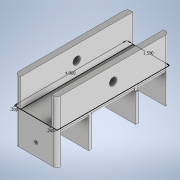
# Autodesk Inventor part: Sample Holder end for 8020-thruhole-widestance-long
Saved by Autodesk Inventor 2020 (Build 240168000, 168)
## iProperties
Created: 2022-02-15
Part Number: Sample Holder end for 8020-thruhole-widestance-long
Material: Generic
Document SubType Name: Modeling
Designer: Beaucage
Density: 1 g/cm^3
Appearance: Default
Author: Beaucage
Autodesk Inventor part; units mm, degrees
ref_plane "YZ Plane" through (0, 0, 0) normal (1, 0, 0) x (0, 1, 0)
ref_plane "XZ Plane" through (0, 0, 0) normal (0, 1, 0) x (-1, 0, 0)
ref_plane "XY Plane" through (0, 0, 0) normal (0, 0, 1) x (1, 0, 0)
sketch "Sketch1" plane through (0, 0, 0) normal (0, 1, 0) x (-1, 0, 0)
  line L0 (0, 0) -> (38.1, 0)
  line L1 (38.1, 0) -> (38.1, -101.6)
  line L2 (38.1, -101.6) -> (0, -101.6)
  line L3 (0, -101.6) -> (0, 0)
  line L4 (38.1, -101.6) -> (33.02, -101.6)
  line L5 (33.02, -101.6) -> (33.02, 0)
  line L6 (33.02, 0) -> (38.1, 0)
  line L7 (38.1, 0) -> (38.1, -101.6)
  line L8 (0, -101.6) -> (5.08, -101.6)
  line L9 (5.08, -101.6) -> (5.08, 0)
  line L10 (5.08, 0) -> (0, 0)
  line L11 (0, 0) -> (0, -101.6)
  dimension "d0" = 38.1
  dimension "d1" = 101.6
  dimension "d2" = 5.08
  dimension "d3" = 5.08
  constraints: 24 end point, 6 parallel, 3 horizontal, 3 perpendicular, 2 point on line
  measures "d0" distance of L1.end L2.end
  measures "d1" distance of L0.end L1.end
  measures "d2" distance of L5.end L6.end
  measures "d3" distance of L10.end L9.end
extrude "Extrusion1" add sketch "Sketch1" along normal blind 25.4 contours L0 L9 L2 L3 | L0 L1 L2 L5
extrude "Extrusion2" add sketch "Sketch1" against normal blind 5.08
sketch "Sketch2" plane through (0, 25.4, 0) normal (1, 0, 0) x (0, 0, -1)
  line L0 (101.6, 0) -> (0, 0) projected
  line L1 (50.8, 0) -> (50.8, -12.7)
  point P0 (0, -25.4)
  dimension "d8" = 12.7
  constraints: 2 end point, 1 midpoint, 1 vertical
  measures "d8" distance of L1.start L1.end
hole "Hole1" at (0, 12.7, -50.8) direction (-1, 0, 0) diameter 6.7564 end through all clearance for "Socket Head Cap Screw" size "1/4" standard "Ansi Unified Screw Threads"
sketch "Sketch3" plane through (0, -5.08, 0) normal (0, -1, 0) x (1, 0, 0)
  line L0 (0, -101.6) -> (-5.08, -101.6) projected
  line L1 (0, -101.6) -> (0, -88.9)
  line L2 (0, 0) -> (0, -101.6) projected
  line L3 (0, -88.9) -> (0, -63.5)
  line L4 (0, -88.9) -> (-19.05, -88.9)
  line L5 (0, -63.5) -> (-19.05, -63.5)
  line L6 (-38.1, -101.6) -> (-38.1, 0) projected
  line L7 (0, -90.4875) -> (-38.1, -90.4875)
  line L8 (-38.1, -90.4875) -> (-38.1, -87.3125)
  line L9 (-38.1, -87.3125) -> (0, -87.3125)
  line L10 (0, -87.3125) -> (0, -90.4875)
  line L11 (0, -90.4875) -> (-38.1, -87.3125) construction
  line L12 (-38.1, -90.4875) -> (0, -87.3125) construction
  line L13 (0, -61.9125) -> (-38.1, -61.9125)
  line L14 (-38.1, -61.9125) -> (-38.1, -65.0875)
  line L15 (-38.1, -65.0875) -> (0, -65.0875)
  line L16 (0, -65.0875) -> (0, -61.9125)
  line L17 (0, -61.9125) -> (-38.1, -65.0875) construction
  line L18 (-38.1, -61.9125) -> (0, -65.0875) construction
  line L19 (-38.1, 0) -> (-38.1, -101.6) projected
  line L20 (-38.1, 0) -> (0, 0)
  line L21 (0, 0) -> (0, -3.175)
  line L22 (0, -3.175) -> (-38.1, -3.175)
  line L23 (-38.1, -3.175) -> (-38.1, 0)
  line L24 (0, -101.6) -> (-38.1, -101.6)
  line L25 (-38.1, -101.6) -> (-38.1, -98.425)
  line L26 (-38.1, -98.425) -> (0, -98.425)
  line L27 (0, -98.425) -> (0, -101.6)
  line L28 (0, -3.175) -> (0, -28.575)
  line L29 (-38.1, -98.425) -> (-38.1, -73.025)
  line L30 (-38.1, -98.425) -> (-12.7, -98.425) construction
  line L31 (0, -28.575) -> (-38.1, -28.575)
  line L32 (-38.1, -28.575) -> (-38.1, -31.115)
  line L33 (-38.1, -31.115) -> (0, -31.115)
  line L34 (0, -31.115) -> (0, -28.575)
  line L35 (-38.1, -73.025) -> (0.7144, -73.025)
  line L36 (0.7144, -73.025) -> (0.7144, -70.485)
  line L37 (0.7144, -70.485) -> (-38.1, -70.485)
  line L38 (-38.1, -70.485) -> (-38.1, -73.025)
  point P0 (0, -65.0875)
  point P1 (0, -61.9125)
  point P2 (0, -87.3125)
  point P3 (-38.1, -90.4875)
  point P4 (0, -90.4875)
  point P5 (0, -98.425)
  point P6 (-38.1, -98.425)
  point P7 (0, -31.115)
  dimension "d16" = 12.7
  dimension "d17" = 25.4
  dimension "d18" = 19.05
  dimension "d19" = 3.175
  dimension "d20" = 3.175
  dimension "d32" = 3.175
  dimension "d33" = 3.175
  dimension "d34" = 25.4
  dimension "d35" = 25.4
  dimension "d36" = 90
  dimension "d37" = 2.54
  dimension "d38" = 2.54
  constraints: 70 end point, 12 parallel, 9 horizontal, 7 perpendicular, 6 point on line, 4 midpoint, 1 collinear, 3 other
  measures "d16" distance of L0.start L1.end
  measures "d17" distance of L1.end L3.end
  measures "d18" distance of L1.end L4.end
  measures "d19" distance of L7.end L8.end
  measures "d20" distance of L14.end L13.end
  measures "d32" distance of L20.end L21.end
  measures "d33" distance of L24.end L25.end
  measures "d34" distance of L21.end L28.end
  measures "d35" distance of L25.end L29.end
  measures "d36" angle of L30 L29
  measures "d37" distance of L32.end L31.end
  measures "d38" distance of L36.end L35.end
extrude "Extrusion3" add sketch "Sketch3" along normal blind 25.4 contours L0 L24 L6 L26 L1 | L35 L6 L37 L2 | L2 L37 L36 L35 | L6 L31 L2 L33 | L6 L20 L2 L22
sketch "Sketch4" plane through (-38.1, -5.08, 0) normal (0, 0, 1) x (1, 0, 0)
  line L0 (38.1, -25.4) -> (19.05, -25.4)
  line L1 (19.05, -25.4) -> (19.05, -13.97)
  point P0 (38.1, 5.08)
  dimension "d23" = 11.43
  constraints: 4 end point, 1 vertical
  measures "d23" distance of L0.end L1.end
hole "Hole2" at (-19.05, -19.05, 0) direction (0, 0, -1) diameter 2.8575 end through all
fillet "Fillet1" radius 3.175 10 edges at (-38.1, -2.54, 0) (0, -2.54, 0) (0, -2.54, -101.6) (-38.1, -2.54, -101.6) (0, -5.08, -85.725) (0, -5.08, -15.875) (0, -5.08, -50.8) (-38.1, -5.08, -85.725) (-38.1, -5.08, -15.875) (-38.1, -5.08, -50.8)
body "Solid1"
